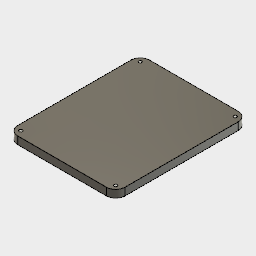
lid v2 (Autodesk Fusion 360 design; units mm, degrees)
Autodesk Fusion 360 part; units mm, degrees
sketch "Sketch1" plane through (0, 0, 0) normal (0, 1, 0) x (1, 0, 0)
  line L0 (0, 0) -> (88.9, 0)
  line L1 (88.9, 0) -> (88.9, -109.22)
  line L2 (88.9, -109.22) -> (0, -109.22)
  line L3 (0, -109.22) -> (0, 0)
  dimension "d1" = 88.9
  dimension "d2" = 109.22
  measures "d1" distance of L0.start L0.end
  measures "d2" distance of L0.start L2.end
extrude "Extrude1" add sketch "Sketch1" along normal blind 6.35
fillet "Fillet1" radius 7.62 4 edges at (88.9, 3.175, 0) (0, 3.175, 0) (88.9, 3.175, 109.22) (0, 3.175, 109.22)
sketch "Sketch2" plane through (0, 6.35, 0) normal (0, 1, 0) x (-1, 0, 0)
  arc A0 (0, 101.6) -> (-7.62, 109.22) centre (-7.62, 101.6) ccw
  line L0 (-7.62, 109.22) -> (-81.28, 109.22)
  arc A1 (-81.28, 109.22) -> (-88.9, 101.6) centre (-81.28, 101.6) ccw
  line L1 (-88.9, 101.6) -> (-88.9, 7.62)
  arc A2 (-88.9, 7.62) -> (-81.28, 0) centre (-81.28, 7.62) ccw
  line L2 (-81.28, 0) -> (-7.62, 0)
  arc A3 (-7.62, 0) -> (0, 7.62) centre (-7.62, 7.62) ccw
  line L3 (0, 7.62) -> (0, 101.6)
  line L4 (-63.8008, 109.22) -> (-63.8008, 101.6)
  line L5 (-88.9, 94.0515) -> (-81.28, 94.0515)
  line L6 (-81.28, 101.6) -> (-7.62, 101.6)
  line L7 (-7.62, 101.6) -> (-7.62, 7.62)
  line L8 (-7.62, 7.62) -> (-81.28, 7.62)
  line L9 (-81.28, 7.62) -> (-81.28, 101.6)
  line L10 (-7.62, 7.62) -> (-5.08, 5.08)
hole "Hole1" at (5.08, 6.35, 5.08) direction (0, -1, 0) diameter 3.175 end through all
sketch "Sketch3" plane through (0, 6.35, 0) normal (0, 1, 0) x (-1, 0, 0)
  circle A0 centre (-5.08, 5.08) radius 1.5875
  arc A1 (0, 101.6) -> (-7.62, 109.22) centre (-7.62, 101.6) ccw
  line L0 (-7.62, 109.22) -> (-81.28, 109.22)
  arc A2 (-81.28, 109.22) -> (-88.9, 101.6) centre (-81.28, 101.6) ccw
  line L1 (-88.9, 101.6) -> (-88.9, 7.62)
  arc A3 (-88.9, 7.62) -> (-81.28, 0) centre (-81.28, 7.62) ccw
  line L2 (-81.28, 0) -> (-7.62, 0)
  arc A4 (-7.62, 0) -> (0, 7.62) centre (-7.62, 7.62) ccw
  line L3 (0, 7.62) -> (0, 101.6)
  line L4 (-50.8, 0) -> (-50.8, 7.62)
  line L5 (-88.9, 22.8139) -> (-81.28, 22.8139)
  line L6 (-81.28, 7.62) -> (-7.62, 7.62)
  line L7 (-7.62, 7.62) -> (-7.62, 101.6)
  line L8 (-7.62, 101.6) -> (-81.28, 101.6)
  line L9 (-81.28, 101.6) -> (-81.28, 7.62)
  line L10 (-81.28, 7.62) -> (-83.82, 5.08)
  line L11 (-7.62, 101.6) -> (-5.08, 104.14)
  line L12 (-81.28, 101.6) -> (-83.82, 104.14)
hole "Hole2" at (83.82, 6.35, 5.08) direction (0, -1, 0) diameter 3.175 end through all
sketch "Sketch4" plane through (0, 6.35, 0) normal (0, 1, 0) x (-1, 0, 0)
  circle A0 centre (-83.82, 5.08) radius 1.5875
  circle A1 centre (-5.08, 5.08) radius 1.5875
  arc A2 (0, 101.6) -> (-7.62, 109.22) centre (-7.62, 101.6) ccw
  line L0 (-7.62, 109.22) -> (-81.28, 109.22)
  arc A3 (-81.28, 109.22) -> (-88.9, 101.6) centre (-81.28, 101.6) ccw
  line L1 (-88.9, 101.6) -> (-88.9, 7.62)
  arc A4 (-88.9, 7.62) -> (-81.28, 0) centre (-81.28, 7.62) ccw
  line L2 (-81.28, 0) -> (-7.62, 0)
  arc A5 (-7.62, 0) -> (0, 7.62) centre (-7.62, 7.62) ccw
  line L3 (0, 7.62) -> (0, 101.6)
  line L4 (0, 73.66) -> (-7.62, 73.66)
  line L5 (-28.8405, 109.22) -> (-28.8405, 101.6)
  line L6 (-7.62, 101.6) -> (-81.28, 101.6)
  line L7 (-81.28, 101.6) -> (-81.28, 60.96)
  line L8 (-81.28, 60.96) -> (-7.62, 60.96)
  line L9 (-7.62, 60.96) -> (-7.62, 101.6)
  line L10 (-44.45, 60.96) -> (-44.45, 101.6)
  line L11 (-7.62, 101.6) -> (-5.08, 104.14)
  line L12 (-81.28, 101.6) -> (-83.82, 104.14)
  point P0 (-83.82, 104.14)
  point P1 (-5.08, 104.14)
hole "Hole3" at (5.08, 6.35, 104.14) at (83.82, 6.35, 104.14) direction (0, -1, 0) diameter 3.175 end through all
thread "Thread1" "ANSI Unified Screw Threads 0.125(#5) 5-40 UNC 3B" major diameter 3.175 minor diameter 2.5933 pitch 0.635 angle 60 resizes the face on face at (5.2381, 4.2333, 6.6596) on face at (84.1346, 4.2333, 6.636) on face at (5.2381, 4.2333, 105.7196) on face at (84.2117, 4.2333, 102.6016)
